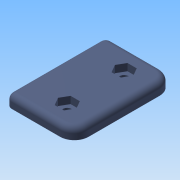
# Autodesk Inventor part: крепление  магнитного замка
Saved by Autodesk Inventor 2017 (Build 210142000, 142)
## iProperties
Part Number: крепление  магнитного замка
Material: Типовые
Document SubType Name: Modeling
Designer: chucha
Density: 1 g/cm^3
Appearance: Резина — синяя
Mass: 3.05952 g
Surface Area: 21.0217 cm^2
Volume: 3.05952 cm^3
Author: chucha
Autodesk Inventor part; units mm, degrees
ref_plane "YZ Plane" through (0, 0, 0) normal (1, 0, 0) x (0, 1, 0)
ref_plane "XZ Plane" through (0, 0, 0) normal (0, 1, 0) x (-1, 0, 0)
ref_plane "XY Plane" through (0, 0, 0) normal (0, 0, 1) x (1, 0, 0)
sketch "Эскиз1" plane through (0, 0, 0) normal (0, 0, 1) x (1, 0, 0)
  line L0 (-178.396, -16.0989) -> (-159.396, -16.0989)
  arc A0 (-159.396, -16.0989) -> (-154.396, -11) centre (-159.395, -11.0989) ccw
  line L1 (-154.396, -11) -> (-154.396, 13.9011)
  arc A1 (-154.396, 13.9011) -> (-159.396, 18.9011) centre (-159.396, 13.9011) ccw
  line L2 (-159.396, 18.9011) -> (-178.396, 18.9011)
  circle A2 centre (-164.396, 11.4011) radius 1.5
  circle A3 centre (-164.396, -8.5989) radius 1.5
  line L3 (-178.396, -16.0989) -> (-178.396, 18.9011)
  point P0 (0, 0)
  dimension "d9" = 20
  dimension "d10" = 7.5
  dimension "d11" = 7.5
  dimension "d12" = 14
  dimension "d13" = 10
  dimension "d14" = 5
  dimension "d15" = 5
  dimension "d16" = 14
  dimension "d17" = 3
  dimension "d18" = 3
  constraints: 8 end point, 4 centre point, 4 point on circle, 2 parallel, 2 tangent
  measures "d9" distance of A3.centre A2.centre
  measures "d10" distance from line of L2 A2.centre
  measures "d11" distance from line of L0 A3.centre
  measures "d12" distance from line of A3.centre L3
  measures "d13" distance from line of L1 A3.centre
  measures "d14" radius of A0
  measures "d15" radius of A1
  measures "d16" distance from line of L3 A2.centre
  measures "d17" diameter of A2
  measures "d18" diameter of A3
extrude "Выдавливание1" add sketch "Эскиз1" along normal blind 4
sketch "Эскиз2" plane through (0, 0, 4) normal (0, 0, 1) x (1, 0, 0)
  circle A0 centre (-164.396, -8.5989) radius 1.5 projected
  circle A1 centre (-164.396, 11.4011) radius 1.5 projected
  line L0 (-178.396, -16.0989) -> (-159.396, -16.0989) projected
  arc A2 (-159.396, -16.0989) -> (-154.396, -11) centre (-159.395, -11.0989) ccw projected
  line L1 (-154.396, -11) -> (-154.396, 13.9011) projected
  arc A3 (-154.396, 13.9011) -> (-159.396, 18.9011) centre (-159.396, 13.9011) ccw projected
  line L2 (-159.396, 18.9011) -> (-178.396, 18.9011) projected
  line L3 (-178.396, 18.9011) -> (-178.396, -16.0989) projected
  circle A4 centre (-164.396, -8.5989) radius 1.5 projected
  line L4 (-167.6291, -8.5989) -> (-166.0125, -5.7989)
  line L5 (-166.0125, -5.7989) -> (-162.7794, -5.7989)
  line L6 (-162.7794, -5.7989) -> (-161.1628, -8.5989)
  line L7 (-161.1628, -8.5989) -> (-162.7794, -11.3989)
  line L8 (-162.7794, -11.3989) -> (-166.0125, -11.3989)
  line L9 (-166.0125, -11.3989) -> (-167.6291, -8.5989)
  line L10 (-167.6291, 11.4011) -> (-166.0125, 14.2011)
  line L11 (-166.0125, 14.2011) -> (-162.7794, 14.2011)
  line L12 (-162.7794, 14.2011) -> (-161.1628, 11.4011)
  line L13 (-161.1628, 11.4011) -> (-162.7794, 8.6011)
  line L14 (-162.7794, 8.6011) -> (-166.0125, 8.6011)
  line L15 (-166.0125, 8.6011) -> (-167.6291, 11.4011)
  line L16 (-159.396, 18.9011) -> (-178.396, 18.9011) projected
  line L17 (-178.396, -16.0989) -> (-159.396, -16.0989) projected
  point P0 (0, 0)
  point P1 (-164.396, 11.4011)
  dimension "d4" = 5.6
  dimension "d5" = 5.6
  constraints: 24 end point, 2 coincident, 2 parallel, 26 other
  measures "d4" distance between parallel lines of L8 L5
  measures "d5" distance between parallel lines of L11 L14
extrude "Выдавливание2" cut sketch "Эскиз2" against normal blind 2.5 contours L4 L5 L6 L7 L8 L9 | L10 L11 L12 L13 L14 L15
fillet "Сопряжение1" radius 2 8 edges at (-178.396, 1.4011, 4) (-155.825, -14.5996, 4) (-154.396, 1.4506, 4) (-155.8604, 17.4367, 4) (-168.896, 18.9011, 4) (-168.896, -16.0989, 4) (-178.396, -16.0989, 2) (-178.396, 18.9011, 2)
